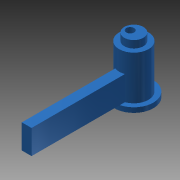
# Autodesk Inventor part: spacer off center
Saved by Autodesk Inventor 2013 (Build 170138000, 138)
## iProperties
Created: 2017-01-26
Part Number: spacer off center
Material: Generic
Document SubType Name: Modeling
Designer: Herman de Vries
Density: 1 g/cm^3
Author: Herman de Vries
Autodesk Inventor part; units mm, degrees
ref_plane "YZ Plane" through (0, 0, 0) normal (1, 0, 0) x (0, 1, 0)
ref_plane "XZ Plane" through (0, 0, 0) normal (0, 1, 0) x (-1, 0, 0)
ref_plane "XY Plane" through (0, 0, 0) normal (0, 0, 1) x (1, 0, 0)
sketch "Sketch1" plane through (0, 0, 0) normal (0, 0, 1) x (1, 0, 0)
  circle A0 centre (0, 0) radius 6
  circle A1 centre (-1.5, 0) radius 1.6
  dimension "d1" = 12
  dimension "d8" = 3.2
  dimension "d9" = 1.5
  constraints: 2 centre point, 1 horizontal alignment
  measures "d1" diameter of A0
  measures "d8" diameter of A1
  measures "d9" distance of A1.centre point (0, 0)
extrude "Extrusion1" add sketch "Sketch1" along normal blind 20
sketch "Sketch2" plane through (0, 0, 20) normal (0, 0, 1) x (1, 0, 0)
  circle A0 centre (0, 0) radius 3.9
  circle A1 centre (-1.5, 0) radius 1.6 projected
  dimension "d4" = 7.8
  constraints: 1 centre point
  measures "d4" diameter of A0
extrude "Extrusion2" add sketch "Sketch2" along normal blind 3
sketch "Sketch3" plane through (0, 0, 0) normal (0, 0, -1) x (-1, 0, 0)
  circle A0 centre (0, 0) radius 8
  circle A1 centre (0, 0) radius 6 projected
  dimension "d10" = 16
  constraints: 1 centre point, 1 coincident
  measures "d10" diameter of A0
extrude "Extrusion3" add sketch "Sketch3" against normal blind 2
sketch "Sketch5" plane through (0, 0, 0) normal (1, 0, 0) x (0, 1, 0)
  line L0 (-44, 2) -> (-4, 2)
  line L1 (-4, 2) -> (-4, 12)
  line L2 (-4, 12) -> (-44, 12)
  line L3 (-44, 12) -> (-44, 2)
  line L4 (-8, 0) -> (8, 0) projected
  line L5 (-8, 0) -> (-8, 2) projected
  point P0 (0, 0)
  dimension "d22" = 40
  dimension "d24" = 10
  dimension "d25" = 4
  dimension "d26" = 0
  constraints: 8 end point, 2 parallel, 1 horizontal, 1 perpendicular
  measures "d22" distance of L1.end L2.end
  measures "d24" distance of L2.end L0.start
  measures "d25" distance from line of L1 L4.start
  measures "d26" distance from line of L5.end L0
extrude "Extrusion5" add sketch "Sketch5" along normal mid plane 4
body "Solid1"
